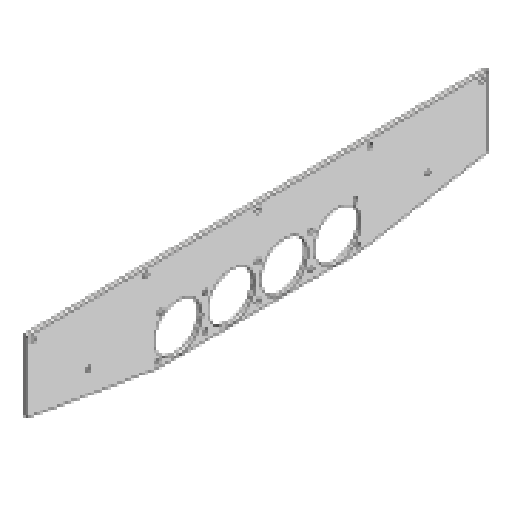
# Autodesk Inventor part: ChassiInsidePlate3.3
Saved by Autodesk Inventor 2023 (Build 270158000, 158)
## iProperties
Created: 2022-11-07
Part Number: ChassiInsidePlate3.3
Material: Generic
Document SubType Name: Modeling
Designer: deli
Density: 1 g/cm^3
Appearance: Default
Author: deli
Autodesk Inventor part; units mm, degrees
ref_plane "YZ Plane" through (0, 0, 0) normal (1, 0, 0) x (0, 1, 0)
ref_plane "XZ Plane" through (0, 0, 0) normal (0, 1, 0) x (-1, 0, 0)
ref_plane "XY Plane" through (0, 0, 0) normal (0, 0, 1) x (1, 0, 0)
sketch "Sketch1" plane through (0, 0, 0) normal (1, 0, 0) x (0, 1, 0)
  arc A0 (526.6307, -141.5559) -> (525.5822, -138.929) centre (524.793, -140.7667) ccw projected
  arc A1 (218.0959, -5.5727) -> (219.3067, -7.4104) centre (220.0959, -5.5727) ccw projected
  line L0 (218.0959, -5.5727) -> (218.0959, 224.2016) projected
  line L1 (218.0959, 224.2016) -> (132.4959, 224.2016) projected
  line L2 (132.4959, 224.2016) -> (114.1693, 118.4948) projected
  arc A2 (114.1693, 118.4948) -> (114.0959, 117.6406) centre (119.0959, 117.6406) ccw projected
  arc A3 (114.0959, -46.9375) -> (114.1693, -47.7916) centre (119.0959, -46.9375) ccw projected
  line L3 (114.1693, -47.7916) -> (132.4959, -153.4984) projected
  line L4 (132.4959, -153.4984) -> (218.0959, -153.4984) projected
  circle A4 centre (185.0959, -148.4984) radius 2 projected
  circle A5 centre (185.0959, 127.2766) radius 2 projected
  circle A6 centre (152.9228, 115.1595) radius 2 projected
  circle A7 centre (152.9228, -44.4563) radius 2 projected
  circle A8 centre (142.0959, 174.2016) radius 2 projected
  circle A9 centre (142.0959, -103.4984) radius 2 projected
  circle A10 centre (134.8459, 100.538) radius 4 projected
  circle A11 centre (134.8459, -29.8348) radius 4 projected
  circle A12 centre (148.4817, -7.9916) radius 2 projected
  circle A13 centre (121.21, -7.9916) radius 2 projected
  circle A14 centre (185.0959, 219.2016) radius 2 projected
  circle A15 centre (185.0959, -56.5734) radius 2 projected
  circle A16 centre (185.0959, 35.3516) radius 2 projected
  circle A17 centre (119.0959, 117.6406) radius 2 projected
  circle A18 centre (119.0959, -46.9375) radius 2 projected
  line L5 (190.0959, 224.2016) -> (190.0959, -153.4984)
  circle A19 centre (134.8459, 100.538) radius 19.5
  circle A20 centre (134.8459, -29.8348) radius 19.5
  line L6 (525.5822, -138.929) -> (506.9866, -130.9439) projected
  line L7 (114.0959, 117.6406) -> (114.0959, -46.9375) projected
  line L8 (218.0959, -153.4984) -> (524.6579, -146.1502) projected
  line L9 (524.6579, -146.1502) -> (526.6307, -141.5559) projected
  circle A21 centre (257.2709, -27.5218) radius 1 projected
  circle A22 centre (339.9687, -63.0333) radius 1 projected
  circle A23 centre (436.4496, -104.4634) radius 1 projected
  circle A24 centre (519.1474, -139.9749) radius 1 projected
  arc A25 (504.4897, -124.6886) -> (506.9866, -130.9439) centre (508.8658, -126.5678) ccw projected
  line L10 (504.4897, -124.6886) -> (507.7005, -117.2113) projected
  arc A26 (507.7005, -117.2113) -> (502.1873, -114.8439) centre (504.9439, -116.0276) ccw projected
  line L11 (502.1873, -114.8439) -> (498.9765, -122.3212) projected
  arc A27 (492.7213, -124.8181) -> (498.9765, -122.3212) centre (494.6004, -120.442) ccw projected
  line L12 (492.7213, -124.8181) -> (219.3067, -7.4104) projected
  circle A28 centre (504.9439, -116.0276) radius 1.5 projected
  circle A29 centre (200.5959, 172.0016) radius 1.6 projected
  circle A30 centre (215.5959, 162.0016) radius 1.6 projected
  circle A31 centre (215.5959, 190.9016) radius 1.6 projected
  circle A32 centre (200.5959, 200.9016) radius 1.6 projected
  circle A33 centre (215.5959, 200.9016) radius 1.6 projected
  circle A34 centre (200.5959, 190.9016) radius 1.6 projected
  circle A35 centre (215.5959, 172.0016) radius 1.6 projected
  circle A36 centre (200.5959, 162.0016) radius 1.6 projected
  circle A37 centre (121.21, 78.6948) radius 2 projected
  circle A38 centre (120.675, 35.3516) radius 2 projected
  circle A39 centre (134.8459, 13.8516) radius 4 projected
  circle A40 centre (134.8459, 56.8516) radius 4 projected
  circle A41 centre (149.0167, 35.3516) radius 2 projected
  circle A42 centre (148.4817, 78.6948) radius 2 projected
  circle A43 centre (134.8459, 56.8516) radius 19.5
  circle A44 centre (134.8459, 13.8516) radius 19.5
  point P0 (0, 0)
  point P1 (114.0959, 111.4062)
  dimension "d0" = 5
  dimension "d1" = 39
  constraints: 4 centre point, 4 coincident, 3 equal radius, 2 end point, 2 point on line, 1 vertical
  measures "d0" distance from line of L5 A5.centre
  measures "d1" diameter of A19
extrude "Extrusion1" add sketch "Sketch1" along normal blind 3.175 contours L4 L3 A3 L7 A2 L2 L1 L5
body "Solid1"
